Stepper NEMA23 10.1kgcm_v1 (Autodesk Fusion 360 design; units mm, degrees)
Autodesk Fusion 360 part; units mm, degrees
sketch "Sketch1" plane through (0, 0, 0) normal (0, 0, 1) x (1, 0, 0)
  line L0 (28.5, -28.5) -> (-28.5, -28.5)
  line L1 (-28.5, -28.5) -> (-28.5, 28.5)
  line L2 (-28.5, 28.5) -> (28.5, 28.5)
  line L3 (28.5, 28.5) -> (28.5, -28.5)
  line L4 (28.5, -28.5) -> (-28.5, 28.5) construction
  line L5 (-28.5, -28.5) -> (28.5, 28.5) construction
  dimension "d1" = 57
  dimension "d2" = 57
  constraint horizontal L0
  constraint perpendicular L0 L1
  constraint parallel L0 L2
  constraint parallel L1 L3
  constraint coincident L4 origin
  constraint coincident L5 origin
  measures "d1" distance of L1.end L2.end
  measures "d2" distance of L0.start L2.end
extrude "Extrude1" add sketch "Sketch1" along normal blind 51
chamfer "Chamfer1" distance 5 angle 45 4 edges at (-28.5, -28.5, 25.5) (28.5, -28.5, 25.5) (-28.5, 28.5, 25.5) (28.5, 28.5, 25.5)
sketch "Sketch2" plane through (0, 0, 51) normal (0, 0, 1) x (-1, 0, 0)
  line L0 (-28.5, -23.5) -> (-23.5, -28.5)
  line L1 (-23.5, -28.5) -> (23.5, -28.5)
  line L2 (23.5, -28.5) -> (28.5, -23.5)
  line L3 (28.5, -23.5) -> (28.5, 23.5)
  line L4 (28.5, 23.5) -> (23.5, 28.5)
  line L5 (23.5, 28.5) -> (-23.5, 28.5)
  line L6 (-23.5, 28.5) -> (-28.5, 23.5)
  line L7 (-28.5, 23.5) -> (-28.5, -23.5)
  circle A0 centre (0, 0) radius 12.5
  circle A1 centre (0, 0) radius 3.175
  dimension "d6" = 25
  dimension "d7" = 6.35
  constraint coincident A0.centre A1.centre
  constraint concentric A0 A1
  measures "d6" diameter of A0
  measures "d7" diameter of A1
extrude "Extrude2" add sketch "Sketch2" along normal blind 2 contours A0
extrude "Extrude3" add 1 faces at (1.0904, 0.6963, 51) along direction (0, 0, 1) blind 20.6
